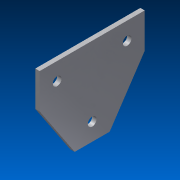
# Autodesk Inventor part: Mounting
Saved by Autodesk Inventor 2013 (Build 170138000, 138)
## iProperties
Created: 2013-07-19
Part Number: Mounting
Material: Aluminum 6061
Document SubType Name: Modeling
Designer: nowireless
Density: 1 g/cm^3
Author: nowireless
Autodesk Inventor part; units mm, degrees
ref_plane "YZ Plane" through (0, 0, 0) normal (1, 0, 0) x (0, 1, 0)
ref_plane "XZ Plane" through (0, 0, 0) normal (0, 1, 0) x (-1, 0, 0)
ref_plane "XY Plane" through (0, 0, 0) normal (0, 0, 1) x (1, 0, 0)
sketch "Sketch1" plane through (0, 0, 0) normal (1, 0, 0) x (0, 1, 0)
  line L0 (0, 0) -> (0, -25.4)
  line L1 (0, -25.4) -> (38.1, -50.8)
  line L2 (38.1, -50.8) -> (63.5, -50.8)
  line L3 (63.5, -50.8) -> (63.5, 25.4)
  line L4 (63.5, 25.4) -> (38.1, 25.4)
  line L5 (38.1, 25.4) -> (0, 0)
  dimension "d0" = 76.2
  dimension "d2" = 25.4
  dimension "d3" = 25.4
  dimension "d4" = 25.4
  dimension "d5" = 63.5
  dimension "d6" = 25.4
  constraints: 12 end point, 2 parallel, 1 perpendicular, 1 vertical
  measures "d0" distance of L2.end L3.end
  measures "d2" distance of L3.end L4.end
  measures "d3" distance of L1.end L2.end
  measures "d4" distance of L0.start L0.end
  measures "d5" distance between parallel lines of L0 L3
  measures "d6" distance from line of L4 L0.start
extrude "Extrusion1" add sketch "Sketch1" along normal blind 3.175
sketch "Sketch2" plane through (3.175, 0, 0) normal (1, 0, 0) x (0, 0, -1)
  line L0 (0, 0) -> (25.4, 0) projected
  line L1 (50.8, 38.1) -> (50.8, 63.5) projected
  line L2 (50.8, 63.5) -> (-25.4, 63.5) projected
  line L3 (-25.4, 63.5) -> (-25.4, 38.1) projected
  point P0 (-12.7, 50.8)
  point P1 (38.1, 50.8)
  point P2 (12.7, 12.7)
  dimension "d9" = 12.7
  dimension "d10" = 12.7
  dimension "d11" = 12.7
  dimension "d12" = 12.7
  dimension "d13" = 12.7
  dimension "d14" = 12.7
  measures "d9" distance from line of point (-12.7, 50.8) L3
  measures "d10" distance from line of point (38.1, 50.8) L1
  measures "d11" distance from line of point (38.1, 50.8) L2
  measures "d12" distance from line of point (-12.7, 50.8) L2
  measures "d13" distance from line of point (12.7, 12.7) L0
  measures "d14" horizontal distance of L0.end point (12.7, 12.7)
hole "Hole1" at (3.175, 50.8, 12.7) at (3.175, 50.8, -38.1) at (3.175, 12.7, -12.7) direction (-1, 0, 0) diameter 6.35 end through all
body "Solid1"
